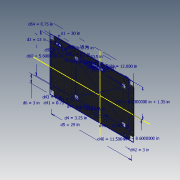
# Autodesk Inventor part: FLUGGER PRESS BASE
Saved by Autodesk Inventor 2020.3 (Build 243373000, 373)
## iProperties
RuleStatus: InUse
AfterDocSave0: file://Part Number Cleaner
Created: 2019-09-30
Material: ACETAL COPOLYMER, BLACK
Vendor: HHMI: JRC - ID&F
Document SubType Name: Modeling
Designer: arnoldj
Density: 1.42 g/cm^3
Appearance: Black Anodize
LAB/DEPT: A. LEE (LAB)
DESIGN DEPARTMENT: HHMI: JRC - ID&F
ALTERED ITEM PART NUMBER: N/A
ALTERED ITEM VENDOR: N/A
ALTERED ITEM DESCRIPTION: N/A
Author: arnoldj
Revision Number: 0
Autodesk Inventor part; units mm, degrees
ref_plane "YZ Plane" through (0, 0, 0) normal (1, 0, 0) x (0, 1, 0)
ref_plane "XZ Plane" through (0, 0, 0) normal (0, 1, 0) x (-1, 0, 0)
ref_plane "XY Plane" through (0, 0, 0) normal (0, 0, 1) x (1, 0, 0)
sketch "Sketch1" plane through (0, 0, 0) normal (0, 0, 1) x (1, 0, 0)
  line L0 (0, 356.108) -> (0, -314.198) projected
  line L1 (-609.6, 0) -> (457.2, 0) projected
  line L2 (304.8, -218.44) -> (-457.2, -218.44)
  line L3 (-457.2, -218.44) -> (-457.2, 260.35)
  line L4 (-457.2, 260.35) -> (304.8, 260.35)
  line L5 (304.8, 260.35) -> (304.8, -218.44)
  line L6 (260.35, -135.89) -> (-260.35, -135.89) construction
  line L7 (-260.35, -135.89) -> (-260.35, 194.31) construction
  line L8 (-260.35, 194.31) -> (260.35, 194.31) construction
  line L9 (260.35, 194.31) -> (260.35, -135.89) construction
  line L10 (260.35, -135.89) -> (-260.35, 194.31) construction
  line L11 (-260.35, -135.89) -> (260.35, 194.31) construction
  line L12 (292.1, -142.24) -> (-444.5, -142.24) construction
  line L13 (-444.5, -142.24) -> (-444.5, 142.24) construction
  line L14 (-444.5, 142.24) -> (292.1, 142.24) construction
  line L15 (292.1, 142.24) -> (292.1, -142.24) construction
  line L16 (215.9, -123.19) -> (-215.9, -123.19) construction
  line L17 (-215.9, -123.19) -> (-215.9, 181.61) construction
  line L18 (-215.9, 181.61) -> (215.9, 181.61) construction
  line L19 (215.9, 181.61) -> (215.9, -123.19) construction
  line L20 (215.9, -123.19) -> (-215.9, 181.61) construction
  line L21 (-215.9, -123.19) -> (215.9, 181.61) construction
  line L22 (76.2, -135.89) -> (-76.2, -135.89) construction
  line L23 (-76.2, -135.89) -> (-76.2, -167.64) construction
  line L24 (-76.2, -167.64) -> (76.2, -167.64) construction
  line L25 (76.2, -167.64) -> (76.2, -135.89) construction
  line L26 (76.2, -135.89) -> (-76.2, -167.64) construction
  line L27 (-76.2, -135.89) -> (76.2, -167.64) construction
  point P0 (0, 0)
  point P1 (0, 29.21)
  point P2 (0, 0)
  point P3 (228.6, -199.39)
  point P4 (-381, -199.39)
  point P5 (-76.2, -199.39)
  point P6 (0, -151.765)
  point P7 (-381, 241.3)
  point P8 (-76.2, 241.3)
  point P9 (228.6, 241.3)
  dimension "d1" = 762
  dimension "d2" = 520.7
  dimension "d3" = 330.2
  dimension "d4" = 82.55
  dimension "d5" = 736.6
  dimension "d6" = 76.2
  dimension "d28" = 431.8
  dimension "d29" = 304.8
  dimension "d38" = 304.8
  dimension "d39" = 260.35
  dimension "d40" = 292.1
  dimension "d41" = 19.05
  dimension "d42" = 76.2
  dimension "d43" = 76.2
  dimension "d44" = 304.8
  dimension "d46" = 304.8
  dimension "d47" = 50.8
  dimension "d48" = 31.75
  dimension "d49" = 152.4
  dimension "d60" = 142.24
  dimension "d61" = 218.44
  dimension "d64" = 19.05
  constraints: 52 end point, 10 coincident, 10 parallel, 6 midpoint, 5 horizontal, 5 perpendicular, 3 horizontal alignment, 3 point on line, 2 vertical alignment
  measures "d1" distance of L3.end L4.end
  measures "d2" distance of L7.end L8.end
  measures "d3" distance of L6.end L7.end
  measures "d4" distance between parallel lines of L6 L2
  measures "d5" distance of L12.start L12.end
  measures "d6" distance between parallel lines of L12 L2
  measures "d28" distance of L17.end L18.end
  measures "d29" distance of L16.end L17.end
  measures "d38" distance between parallel lines of L5 L0
  measures "d39" distance between parallel lines of L4 L1
  measures "d40" distance between parallel lines of L0 L15
  measures "d41" distance from line of L2 point (-381, -199.39)
  measures "d42" distance from line of point (228.6, -199.39) L5
  measures "d43" distance from line of L3 point (-381, -199.39)
  measures "d44" distance of point (-381, -199.39) point (-76.2, -199.39)
  measures "d46" distance of point (228.6, -199.39) point (-76.2, -199.39)
  measures "d47" distance between parallel lines of L24 L2
  measures "d48" distance of L22.end L23.end
  measures "d49" distance of L22.start L22.end
  measures "d60" distance between parallel lines of L1 L14
  measures "d61" distance between parallel lines of L2 L1
  measures "d64" distance from line of point (-381, 241.3) L4
extrude "Extrusion1" add sketch "Sketch1" against normal blind 6.35
hole "Hole1" at (-260.35, 194.31, 0) at (-260.35, -135.89, 0) at (260.35, -135.89, 0) at (260.35, 194.31, 0) direction (0, 0, -1) diameter 9.525 end through all
hole "Hole2" at (-444.5, -142.24, 0) at (-444.5, 142.24, 0) at (292.1, 142.24, 0) at (292.1, -142.24, 0) at (-381, -199.39, 0) at (-76.2, -199.39, 0) at (228.6, -199.39, 0) at (-381, 241.3, 0) at (-76.2, 241.3, 0) at (228.6, 241.3, 0) direction (0, 0, -1) diameter 11.43 end through all
sketch "Sketch2" plane through (0, 0, 0) normal (0, 0, 1) x (1, 0, 0)
  line L0 (-457.2, -218.44) -> (-457.2, 260.35) projected
  line L1 (-457.2, -218.44) -> (-421.64, -218.44)
  line L2 (-421.64, -218.44) -> (-421.64, -177.8)
  line L3 (-421.64, -177.8) -> (-457.2, -177.8)
  line L4 (-457.2, -177.8) -> (-457.2, -218.44)
  line L5 (304.8, -218.44) -> (-457.2, -218.44) projected
  line L6 (304.8, -218.44) -> (269.24, -218.44)
  line L7 (269.24, -218.44) -> (269.24, -177.8)
  line L8 (269.24, -177.8) -> (304.8, -177.8)
  line L9 (304.8, -177.8) -> (304.8, -218.44)
  line L10 (-457.2, 219.71) -> (-421.64, 219.71)
  line L11 (-421.64, 219.71) -> (-421.64, 260.35)
  line L12 (-457.2, 260.35) -> (304.8, 260.35) projected
  line L13 (269.24, 260.35) -> (269.24, 219.71)
  line L14 (269.24, 219.71) -> (304.8, 219.71)
  line L15 (304.8, 260.35) -> (304.8, -218.44) projected
  point P0 (0, 0)
  dimension "d24" = 35.56
  dimension "d37" = 40.64
  dimension "d62" = 35.56
  dimension "d63" = 40.64
  constraints: 24 end point, 5 point on line, 4 parallel, 4 perpendicular, 3 equal length, 3 horizontal, 1 vertical
  measures "d24" distance of L2.end L3.end
  measures "d37" distance of L1.end L2.end
  measures "d62" distance between parallel lines of L0 L11
  measures "d63" distance between parallel lines of L10 L12
extrude "Extrusion2" cut sketch "Sketch2" against normal blind 6.35 contours L0 L3 L2 L1 | L0 L12 L11 L10 | L7 L8 L9 L5 | L12 L15 L14 L13
fillet "Fillet1" radius 6.35 8 edges at (269.24, -218.44, -3.175) (304.8, -177.8, -3.175) (-421.64, -218.44, -3.175) (-457.2, -177.8, -3.175) (-457.2, 219.71, -3.175) (-421.64, 260.35, -3.175) (269.24, 260.35, -3.175) (304.8, 219.71, -3.175)
hole "Hole3" at (-215.9, 181.61, 0) at (215.9, 181.61, 0) at (215.9, -123.19, 0) at (-215.9, -123.19, 0) direction (0, 0, -1) diameter 38.1 end through all
hole "Hole4" at (-76.2, -135.89, 0) at (-76.2, -167.64, 0) direction (0, 0, -1) diameter 3.1242 depth 25.4 tip angle 118
pattern_linear "Rectangular Pattern1" count 4 spacing 50.8 along (1, 0, 0) of "Hole4"
sketch "Sketch3" plane through (0, 0, 0) normal (0, 0, 1) x (1, 0, 0)
  line L0 (0, 356.108) -> (0, -314.198) projected
  line L1 (-609.6, 0) -> (457.2, 0) projected
  line L2 (25.4, 199.39) -> (-25.4, 199.39)
  line L3 (-25.4, 199.39) -> (-25.4, 224.79)
  line L4 (-25.4, 224.79) -> (25.4, 224.79)
  line L5 (25.4, 224.79) -> (25.4, 199.39)
  line L6 (25.4, 199.39) -> (-25.4, 224.79) construction
  line L7 (-25.4, 199.39) -> (25.4, 224.79) construction
  line L8 (-415.29, 260.35) -> (262.89, 260.35) projected
  line L9 (-355.6, 199.39) -> (-406.4, 199.39)
  line L10 (-406.4, 199.39) -> (-406.4, 224.79)
  line L11 (-406.4, 224.79) -> (-355.6, 224.79)
  line L12 (-355.6, 224.79) -> (-355.6, 199.39)
  line L13 (-355.6, 199.39) -> (-406.4, 224.79) construction
  line L14 (-406.4, 199.39) -> (-355.6, 224.79) construction
  line L15 (-25.4, 224.79) -> (-76.2, 224.79)
  line L16 (-76.2, 224.79) -> (-76.2, 199.39)
  line L17 (-76.2, 199.39) -> (-25.4, 199.39)
  line L18 (-25.4, 199.39) -> (-25.4, 224.79)
  point P0 (0, 0)
  point P1 (0, 212.09)
  point P2 (-381, 212.09)
  point P3 (-381, 212.09)
  point P4 (0, 212.09)
  point P5 (-342.9, 212.09)
  point P6 (-419.1, 212.09)
  point P7 (38.1, 224.79)
  point P8 (-38.1, 224.79)
  point P9 (0, 212.09)
  point P10 (-381, 212.09)
  point P11 (-196.85, 224.79)
  point P12 (-215.9, 181.61)
  point P13 (-209.55, 224.79)
  point P14 (-222.25, 224.79)
  point P15 (-234.95, 224.79)
  dimension "d65" = 35.56
  dimension "d66" = 50.8
  dimension "d67" = 25.4
  dimension "d68" = 381
  dimension "d69" = 50.8
  dimension "d91" = 38.1
  dimension "d92" = 38.1
  dimension "d95" = 12.7
  dimension "d96" = 38.1
  dimension "d97" = 38.1
  dimension "d98" = 25.4
  dimension "d99" = 50.8
  dimension "d100" = 19.05
  dimension "d103" = 12.7
  constraints: 32 end point, 8 midpoint, 7 parallel, 4 horizontal, 4 horizontal alignment, 3 perpendicular, 1 point on line, 3 other
  measures "d65" distance between parallel lines of L4 L8
  measures "d66" distance of L3.end L4.end
  measures "d67" distance of L2.end L3.end
  measures "d68" distance from line of L0 point (-381, 212.09)
  measures "d69" distance of L9.start L9.end
  measures "d91" distance of point (-381, 212.09) point (-342.9, 212.09)
  measures "d92" distance of point (-419.1, 212.09) point (-381, 212.09)
  measures "d95" vertical distance of point (0, 212.09) point (-38.1, 224.79)
  measures "d96" distance from line of L0 point (-38.1, 224.79)
  measures "d97" distance from line of point (38.1, 224.79) L0
  measures "d98" distance of L15.end L16.end
  measures "d99" distance of L3.end L15.end
  measures "d100" horizontal distance of point (-215.9, 181.61) point (-196.85, 224.79)
  measures "d103" distance of point (-196.85, 224.79) point (-209.55, 224.79)
extrude "Extrusion3" cut sketch "Sketch3" against normal through all
fillet "Fillet2" radius 3.175 8 edges at (-406.4, 224.79, -3.175) (-355.6, 224.79, -3.175) (-355.6, 199.39, -3.175) (-406.4, 199.39, -3.175) (25.4, 224.79, -3.175) (25.4, 199.39, -3.175) (-76.2, 224.79, -3.175) (-76.2, 199.39, -3.175)
fillet "Fillet3" radius 3.175 4 edges at (-421.64, -177.8, -3.175) (269.24, -177.8, -3.175) (269.24, 219.71, -3.175) (-421.64, 219.71, -3.175)
sketch "Sketch4" plane through (0, 0, 0) normal (0, 0, 1) x (1, 0, 0)
  line L0 (-444.5, -142.24) -> (-444.5, 142.24) construction
  line L1 (292.1, 142.24) -> (292.1, -142.24) construction
  circle A0 centre (292.1, -142.24) radius 5.715 projected
  circle A1 centre (-381, 241.3) radius 5.715 construction
  circle A2 centre (228.6, 241.3) radius 5.715 construction
  line L2 (-381, 241.3) -> (228.6, 241.3) construction
  line L3 (-406.4, -161.29) -> (-304.8, -161.29) construction
  line L4 (-304.8, -161.29) -> (-304.8, -85.09) construction
  line L5 (-304.8, -85.09) -> (-406.4, -85.09) construction
  line L6 (-406.4, -85.09) -> (-406.4, -161.29) construction
  point P0 (0, 0)
  point P1 (-444.5, -66.04)
  point P2 (-444.5, 66.04)
  point P3 (292.1, 66.04)
  point P4 (292.1, -66.04)
  point P5 (292.1, -66.04)
  point P6 (-304.8, 241.3)
  point P7 (152.4, 241.3)
  point P8 (-406.4, -123.19)
  point P9 (-304.8, -123.19)
  point P10 (-381, -199.39)
  point P11 (-355.6, -85.09)
  point P12 (-355.6, -161.29)
  point P13 (-419.1, 212.09)
  point P14 (-342.9, 212.09)
  point P15 (-38.1, 224.79)
  point P16 (38.1, 224.79)
  dimension "d74" = 76.2
  dimension "d75" = 76.2
  dimension "d76" = 76.2
  dimension "d77" = 76.2
  dimension "d85" = 76.2
  dimension "d86" = 76.2
  dimension "d87" = 101.6
  dimension "d88" = 76.2
  dimension "d89" = 38.1
  dimension "d90" = 38.1
  constraints: 10 end point, 6 coincident, 6 point on line, 4 midpoint, 2 horizontal, 2 parallel, 1 perpendicular
  measures "d74" distance of point (292.1, -66.04) point (292.1, -142.24)
  measures "d75" distance of L1.start point (292.1, 66.04)
  measures "d76" distance of L0.end point (-444.5, 66.04)
  measures "d77" distance of point (-444.5, -66.04) L0.start
  measures "d85" distance of L2.start point (-304.8, 241.3)
  measures "d86" distance of L2.end point (152.4, 241.3)
  measures "d87" distance of L4.end L5.end
  measures "d88" distance of L5.end L3.start
  measures "d89" distance from line of L3 point (-381, -199.39)
  measures "d90" distance between parallel lines of L6 L0
hole "Hole5" at (-444.5, 66.04, 0) at (-444.5, -66.04, 0) at (292.1, 66.04, 0) at (292.1, -66.04, 0) at (-406.4, -85.09, 0) at (-355.6, -85.09, 0) at (-304.8, -85.09, 0) at (-304.8, -123.19, 0) at (-304.8, -161.29, 0) at (-355.6, -161.29, 0) at (-406.4, -161.29, 0) at (-406.4, -123.19, 0) at (-419.1, 212.09, 0) at (-342.9, 212.09, 0) at (38.1, 224.79, 0) direction (0, 0, -1) diameter 3.1242 end through all
hole "Hole6" at (-234.95, 224.79, 0) at (-222.25, 224.79, 0) at (-209.55, 224.79, 0) at (-196.85, 224.79, 0) direction (0, 0, -1) diameter 7.9375 end through all
body "Solid1"
